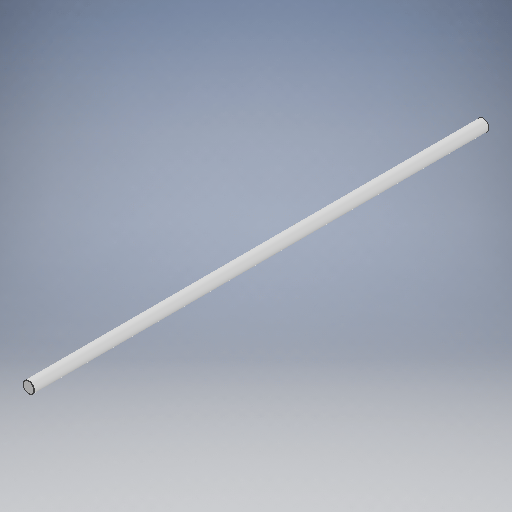
# Autodesk Inventor part: rodshaft_10x400
Saved by Autodesk Inventor 2025.2 (Build 292293000, 293)
## iProperties
Created: 2025-04-06
Part Number: rodshaft_10x400
Material: Generic
Document SubType Name: Modeling
Designer: Tiago
Density: 1 g/cm^3
Appearance: Default
Author: Tiago
Autodesk Inventor part; units mm, degrees
ref_plane "YZ Plane" through (0, 0, 0) normal (1, 0, 0) x (0, 1, 0)
ref_plane "XZ Plane" through (0, 0, 0) normal (0, 1, 0) x (-1, 0, 0)
ref_plane "XY Plane" through (0, 0, 0) normal (0, 0, 1) x (1, 0, 0)
sketch "Sketch1" plane through (0, 0, 0) normal (0, 0, 1) x (1, 0, 0)
  circle A0 centre (0, 0) radius 5
  dimension "Base" = 10
  constraints: 1 centre point, 1 coincident
  measures "Base" diameter of A0
extrude "Extrusion1" add sketch "Sketch1" along normal blind 400
chamfer "Chamfer1" distance 0.3 angle 45 2 edges at (-5, 0, 400) (-5, 0, 0)
body "Solid1"
